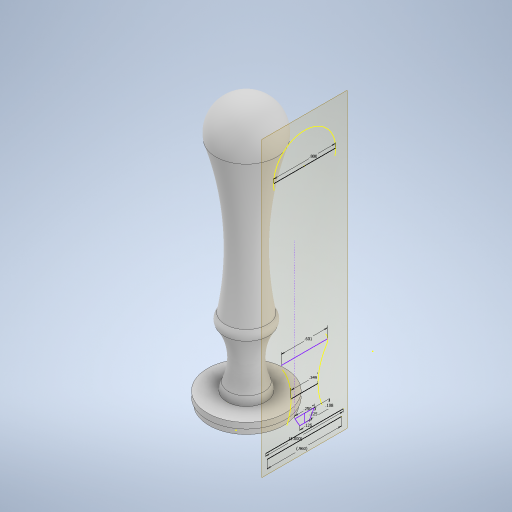
# Autodesk Inventor part: Basic seal 1 full peice
Saved by Autodesk Inventor 2024 (Build 280153000, 153)
## iProperties
Created: 2023-05-18
Part Number: Basic seal 1 full peice
Material: Generic
Document SubType Name: Modeling
Designer: newic
Density: 1 g/cm^3
Appearance: Default
Author: newic
Autodesk Inventor part; units mm, degrees
ref_plane "XZ Plane" through (0, 0, 0) normal (0, 1, 0) x (-1, 0, 0)
ref_plane "XY Plane" through (0, 0, 0) normal (0, 0, 1) x (1, 0, 0)
sketch "Sketch1" plane through (0, 0, 0) normal (0, 1, 0) x (-1, 0, 0)
  circle A0 centre (0, 0) radius 12.7
  line L0 (12.7, 12.7) -> (12.7, -12.7) construction
  line L1 (12.7, -12.7) -> (-12.7, -12.7) construction
  line L2 (-12.7, -12.7) -> (-12.7, 12.7) construction
  line L3 (-12.7, 12.7) -> (12.7, 12.7) construction
  circle A1 centre (0, 0) radius 12.1875
  circle A2 centre (0, 0) radius 11.5722
  line L4 (12.7, 0) -> (-28.224, 0)
  spline S0 degree 4 poles (7.5608, 0) (7.5871, -0.2498) (7.5716, -0.8639) (7.6635, -1.72) (7.771, -2.5827) (7.8796, -3.1444) (8.0283, -3.9996) (8.2528, -4.7367) (8.3389, -5.0369) (8.4927, -5.4299) (8.607, -5.7477) (8.7077, -5.9466) (8.7297, -6.0528) (8.7259, -6.1323) (8.6915, -6.2267) (8.6084, -6.3073) (8.4656, -6.4322) (8.3108, -6.5585) (7.9581, -6.8561) (7.7627, -7.0404) (7.5994, -7.1572) (7.2874, -7.4352) (7.0492, -7.6385) (6.8557, -7.7767) (6.6363, -7.9955) (6.5444, -8.04) (6.425, -8.09) (6.3049, -8.0852) (6.1612, -8.0439) (5.8673, -7.9243) (5.2047, -7.7184) (4.9544, -7.6282) (4.5834, -7.5418) (3.9869, -7.3825) (3.5585, -7.2836) (3.3261, -7.2353) (2.6639, -7.1283) (2.4923, -7.0851) (1.885, -7.0109) (1.2249, -6.9515) (0.9978, -6.9092) (-0.0967, -6.8274) (-0.0908, -6.8879) (-0.9888, -6.8956) (-1.4498, -6.994) (-2.157, -7.03) (-2.8755, -7.1861) (-3.3866, -7.2397) (-4.3934, -7.4794) (-4.8139, -7.612) (-5.3152, -7.7313) (-5.615, -7.8484) (-5.8655, -7.9444) (-6.1746, -8.0443) (-6.2691, -8.0783) (-6.3955, -8.0918) (-6.486, -8.0779) (-6.6705, -8.0058) (-6.661, -7.9168) (-6.8879, -7.7874) (-7.0089, -7.6489) (-7.1824, -7.5178) (-7.3229, -7.3873) (-7.5822, -7.175) (-7.7931, -7.0025) (-8.0826, -6.7466) (-8.2527, -6.613) (-8.4352, -6.4317) (-8.5724, -6.3549) (-8.667, -6.2237) (-8.6858, -6.2037) (-8.7162, -6.092) (-8.7131, -6.0317) (-8.695, -5.9554) (-8.5854, -5.7043) (-8.4697, -5.4626) (-8.3913, -5.2076) (-8.2879, -4.9538) (-8.1958, -4.6121) (-8.0468, -4.045) (-7.9725, -3.8304) (-7.7592, -2.661) (-7.6907, -2.1909) (-7.6151, -1.4373) (-7.564, -0.619) (-7.5516, -0.3428) (-7.5554, -0.0046) (-7.5638, 0) knots 0 0 0 0 0 0.039296 0.055908 0.073069 0.090127 0.10618 0.121509 0.134965 0.146316 0.15619 0.164179 0.170591 0.176443 0.182863 0.190407 0.199969 0.210544 0.221389 0.232964 0.244031 0.25516 0.266564 0.276442 0.284967 0.292352 0.298886 0.30652 0.31685 0.32851 0.341463 0.355682 0.368855 0.381917 0.395666 0.408085 0.420945 0.435034 0.448763 0.464427 0.47884 0.493305 0.508372 0.522986 0.539358 0.555691 0.57306 0.589942 0.605994 0.620829 0.633477 0.645128 0.655027 0.663676 0.671144 0.677933 0.684628 0.692084 0.700281 0.708721 0.71788 0.727519 0.737693 0.74871 0.760009 0.770972 0.781161 0.789961 0.797299 0.803676 0.809144 0.814179 0.820577 0.828361 0.837524 0.847989 0.859019 0.870721 0.882901 0.897625 0.913523 0.930287 0.948149 0.964022 0.978288 1 1 1 1 1
  spline S1 degree 4 poles (7.5608, 0) (7.5871, 0.2498) (7.5716, 0.8639) (7.6635, 1.72) (7.771, 2.5827) (7.8796, 3.1444) (8.0283, 3.9996) (8.2528, 4.7367) (8.3389, 5.0368) (8.4927, 5.4299) (8.607, 5.7477) (8.7077, 5.9466) (8.7297, 6.0528) (8.7259, 6.1323) (8.6915, 6.2267) (8.6084, 6.3073) (8.4656, 6.4322) (8.3108, 6.5585) (7.9581, 6.8561) (7.7627, 7.0404) (7.5994, 7.1572) (7.2874, 7.4352) (7.0492, 7.6385) (6.8557, 7.7767) (6.6363, 7.9955) (6.5444, 8.04) (6.425, 8.09) (6.3049, 8.0852) (6.1612, 8.0439) (5.8673, 7.9243) (5.2047, 7.7184) (4.9544, 7.6282) (4.5834, 7.5418) (3.9869, 7.3825) (3.5585, 7.2836) (3.3261, 7.2353) (2.6639, 7.1283) (2.4923, 7.0851) (1.885, 7.0109) (1.2249, 6.9515) (0.9978, 6.9092) (-0.0967, 6.8274) (-0.0908, 6.8879) (-0.9888, 6.8956) (-1.4498, 6.994) (-2.157, 7.03) (-2.8755, 7.1861) (-3.3866, 7.2397) (-4.3934, 7.4794) (-4.8139, 7.612) (-5.3152, 7.7313) (-5.615, 7.8484) (-5.8655, 7.9444) (-6.1746, 8.0443) (-6.2691, 8.0783) (-6.3955, 8.0918) (-6.486, 8.0779) (-6.6705, 8.0058) (-6.661, 7.9168) (-6.8879, 7.7874) (-7.0089, 7.6489) (-7.1824, 7.5178) (-7.3229, 7.3873) (-7.5822, 7.175) (-7.7931, 7.0025) (-8.0826, 6.7466) (-8.2527, 6.613) (-8.4352, 6.4317) (-8.5724, 6.3549) (-8.667, 6.2237) (-8.6858, 6.2037) (-8.7162, 6.092) (-8.7131, 6.0317) (-8.695, 5.9554) (-8.5854, 5.7043) (-8.4697, 5.4626) (-8.3913, 5.2076) (-8.2879, 4.9538) (-8.1958, 4.6121) (-8.0468, 4.045) (-7.9725, 3.8304) (-7.7592, 2.661) (-7.6907, 2.1909) (-7.6151, 1.4373) (-7.564, 0.619) (-7.5516, 0.3428) (-7.5554, 0.0046) (-7.5638, 0) knots 0 0 0 0 0 0.039296 0.055908 0.073069 0.090127 0.10618 0.121509 0.134965 0.146316 0.15619 0.164179 0.170591 0.176443 0.182863 0.190407 0.199969 0.210544 0.221389 0.232964 0.244031 0.25516 0.266564 0.276442 0.284967 0.292352 0.298886 0.30652 0.31685 0.32851 0.341463 0.355682 0.368855 0.381917 0.395666 0.408085 0.420945 0.435034 0.448763 0.464427 0.47884 0.493305 0.508372 0.522986 0.539358 0.555691 0.57306 0.589942 0.605994 0.620829 0.633477 0.645128 0.655027 0.663676 0.671144 0.677933 0.684628 0.692084 0.700281 0.708721 0.71788 0.727519 0.737693 0.74871 0.760009 0.770972 0.781161 0.789961 0.797299 0.803676 0.809144 0.814179 0.820577 0.828361 0.837524 0.847989 0.859019 0.870721 0.882901 0.897625 0.913523 0.930287 0.948149 0.964022 0.978288 1 1 1 1 1
  spline S2 degree 4 poles (6.6698, 0) (6.6871, -0.3978) (6.6713, -0.7815) (6.7409, -1.5229) (6.8536, -2.5936) (6.9252, -2.906) (7.0997, -3.8444) (7.2267, -4.3825) (7.3633, -4.7956) (7.4896, -5.3512) (7.6112, -5.5391) (7.6677, -5.7689) (7.6975, -5.7897) (7.7062, -5.8965) (7.6285, -5.9815) (7.572, -6.0514) (7.3996, -6.178) (7.1331, -6.4178) (6.9588, -6.5681) (6.6364, -6.8323) (6.5004, -6.9541) (6.3704, -7.0647) (6.3037, -7.1086) (6.2234, -7.1388) (6.1631, -7.1283) (6.0268, -7.0924) (5.9076, -7.0514) (5.5806, -6.952) (5.3855, -6.8908) (5.038, -6.812) (4.9484, -6.7624) (4.2814, -6.6028) (4.0156, -6.5429) (3.8882, -6.5183) (3.3037, -6.3965) (2.8824, -6.3286) (2.5502, -6.2731) (2.4025, -6.2241) (1.6246, -6.1518) (1.37, -6.0874) (1.1134, -6.1) (0.6072, -6.0267) (0.5913, -6.054) (0.1833, -6.0225) (0.0815, -6.0123) (-0.2846, -6.0335) (-0.5883, -6.0362) (-0.9225, -6.0806) (-1.3996, -6.1121) (-1.6329, -6.1378) (-2.1126, -6.197) (-2.4639, -6.2503) (-2.782, -6.3007) (-3.1586, -6.3702) (-3.2077, -6.3787) (-3.7538, -6.4818) (-4.0918, -6.5436) (-4.3482, -6.6242) (-4.8814, -6.7303) (-5.2054, -6.8556) (-5.5087, -6.9063) (-5.6572, -6.9822) (-5.9526, -7.0706) (-6.1139, -7.1317) (-6.1762, -7.1269) (-6.2789, -7.1205) (-6.425, -7.0257) (-6.5484, -6.9167) (-6.706, -6.7703) (-6.9687, -6.5457) (-7.0919, -6.4669) (-7.3885, -6.1958) (-7.4865, -6.1263) (-7.6283, -5.9822) (-7.6822, -5.9316) (-7.7081, -5.8596) (-7.7006, -5.7637) (-7.6112, -5.6344) (-7.5282, -5.3549) (-7.4652, -5.1836) (-7.3295, -4.7829) (-7.1819, -4.1547) (-7.1117, -3.848) (-6.9524, -3.2013) (-6.8781, -2.6524) (-6.8463, -2.4403) (-6.7659, -1.8396) (-6.735, -1.4493) (-6.7089, -1.1731) (-6.6784, -0.6337) (-6.6716, -0.3941) (-6.6731, -0.0474) (-6.6763, 0) knots 0 0 0 0 0 0.039448 0.055349 0.072269 0.088737 0.104506 0.120552 0.134467 0.146293 0.155548 0.162505 0.168442 0.174025 0.180717 0.189099 0.198791 0.210185 0.221737 0.232089 0.240921 0.247815 0.253612 0.259204 0.265359 0.273108 0.282299 0.292472 0.302955 0.314654 0.326295 0.337305 0.349803 0.361846 0.37389 0.386284 0.399242 0.411449 0.423896 0.437159 0.44785 0.458402 0.468238 0.477683 0.488335 0.499312 0.51153 0.523717 0.536339 0.54908 0.561517 0.573881 0.584661 0.595665 0.606838 0.61814 0.631344 0.644301 0.656608 0.668396 0.679342 0.688982 0.697238 0.704622 0.711137 0.717919 0.725945 0.735426 0.745345 0.756153 0.766663 0.776344 0.78489 0.791619 0.7976 0.803458 0.810655 0.819014 0.829148 0.841433 0.854403 0.869138 0.884301 0.898105 0.912368 0.925751 0.938316 0.951323 0.9634 0.975086 1 1 1 1 1
  spline S3 degree 4 poles (6.6698, 0) (6.6871, 0.3978) (6.6713, 0.7814) (6.7409, 1.5229) (6.8536, 2.5936) (6.9252, 2.906) (7.0997, 3.8444) (7.2267, 4.3825) (7.3633, 4.7956) (7.4896, 5.3512) (7.6112, 5.5391) (7.6677, 5.7689) (7.6975, 5.7897) (7.7062, 5.8965) (7.6285, 5.9815) (7.572, 6.0514) (7.3996, 6.178) (7.1331, 6.4178) (6.9588, 6.5681) (6.6364, 6.8323) (6.5004, 6.9541) (6.3704, 7.0646) (6.3037, 7.1085) (6.2234, 7.1388) (6.1631, 7.1283) (6.0268, 7.0924) (5.9076, 7.0514) (5.5806, 6.952) (5.3855, 6.8908) (5.038, 6.812) (4.9484, 6.7624) (4.2814, 6.6028) (4.0156, 6.5429) (3.8882, 6.5183) (3.3037, 6.3965) (2.8824, 6.3286) (2.5502, 6.2731) (2.4025, 6.2241) (1.6246, 6.1517) (1.37, 6.0874) (1.1134, 6.1) (0.6072, 6.0267) (0.5913, 6.054) (0.1833, 6.0225) (0.0815, 6.0123) (-0.2846, 6.0335) (-0.5883, 6.0362) (-0.9225, 6.0806) (-1.3996, 6.1121) (-1.6329, 6.1378) (-2.1126, 6.197) (-2.4639, 6.2503) (-2.782, 6.3007) (-3.1586, 6.3702) (-3.2077, 6.3787) (-3.7538, 6.4818) (-4.0918, 6.5436) (-4.3482, 6.6242) (-4.8814, 6.7303) (-5.2054, 6.8556) (-5.5087, 6.9063) (-5.6572, 6.9822) (-5.9526, 7.0706) (-6.1139, 7.1317) (-6.1762, 7.1269) (-6.2789, 7.1205) (-6.425, 7.0257) (-6.5484, 6.9166) (-6.706, 6.7703) (-6.9687, 6.5457) (-7.0919, 6.4669) (-7.3885, 6.1958) (-7.4865, 6.1263) (-7.6283, 5.9822) (-7.6822, 5.9316) (-7.7081, 5.8596) (-7.7006, 5.7637) (-7.6112, 5.6344) (-7.5282, 5.3549) (-7.4652, 5.1836) (-7.3295, 4.7829) (-7.1819, 4.1547) (-7.1117, 3.848) (-6.9524, 3.2013) (-6.8781, 2.6524) (-6.8463, 2.4403) (-6.7659, 1.8396) (-6.735, 1.4493) (-6.7089, 1.1731) (-6.6784, 0.6337) (-6.6716, 0.3941) (-6.6731, 0.0474) (-6.6763, 0) knots 0 0 0 0 0 0.039448 0.055349 0.072269 0.088737 0.104506 0.120552 0.134467 0.146293 0.155548 0.162505 0.168442 0.174025 0.180717 0.189099 0.198791 0.210185 0.221737 0.232089 0.240921 0.247815 0.253612 0.259204 0.265359 0.273108 0.282299 0.292472 0.302955 0.314654 0.326295 0.337305 0.349803 0.361846 0.37389 0.386284 0.399242 0.411449 0.423896 0.437159 0.44785 0.458402 0.468238 0.477683 0.488335 0.499312 0.51153 0.523717 0.536339 0.54908 0.561517 0.573881 0.584661 0.595665 0.606838 0.61814 0.631344 0.644301 0.656608 0.668396 0.679342 0.688982 0.697238 0.704622 0.711137 0.717919 0.725945 0.735426 0.745345 0.756153 0.766663 0.776344 0.78489 0.791619 0.7976 0.803458 0.810655 0.819014 0.829148 0.841433 0.854403 0.869138 0.884301 0.898105 0.912368 0.925751 0.938316 0.951323 0.9634 0.975086 1 1 1 1 1
  line L5 (1.0941, 0) -> (1.0941, -2.0952)
  line L6 (1.0941, -2.0952) -> (3.9049, -2.2474)
  line L7 (3.9049, -2.2474) -> (4.7904, -1.5612)
  line L8 (-0.5884, 0) -> (-0.5898, -1.9938)
  line L9 (-0.5898, -1.9938) -> (-4.3298, -1.7894)
  line L10 (-4.3298, -1.7894) -> (-5.2324, -1.0809)
  line L11 (5.0927, -1.7005) -> (5.1051, -4.9152)
  line L12 (4.7853, -5.0014) -> (3.8243, -3.9243)
  line L13 (3.8243, -3.9243) -> (-4.2884, -3.485)
  line L14 (-4.2884, -3.485) -> (-5.2324, -4.5455)
  line L15 (-5.5377, -4.4469) -> (-5.5322, -1.2345)
  arc A3 (5.0927, -1.7005) -> (4.7904, -1.5612) centre (4.931, -1.6537) ccw
  arc A4 (4.7853, -5.0014) -> (5.1051, -4.9152) centre (4.9338, -4.9158) ccw
  arc A5 (-5.5377, -4.4469) -> (-5.2324, -4.5455) centre (-5.3693, -4.4472) ccw
  arc A6 (-5.2324, -1.0809) -> (-5.5322, -1.2345) centre (-5.368, -1.1857) ccw
  line L16 (1.0941, 0) -> (1.0941, 2.0952)
  line L17 (1.0941, 2.0952) -> (3.9049, 2.2474)
  line L18 (3.9049, 2.2474) -> (4.7904, 1.5612)
  line L19 (-0.5884, 0) -> (-0.5898, 1.9938)
  line L20 (-0.5898, 1.9938) -> (-4.3298, 1.7894)
  line L21 (-4.3298, 1.7894) -> (-5.2324, 1.0809)
  line L22 (5.0927, 1.7005) -> (5.1051, 4.9152)
  line L23 (4.7853, 5.0014) -> (3.8243, 3.9243)
  line L24 (3.8243, 3.9243) -> (-4.2884, 3.485)
  line L25 (-4.2884, 3.485) -> (-5.2324, 4.5455)
  arc A7 (4.7904, 1.5612) -> (5.0927, 1.7005) centre (4.931, 1.6537) ccw
  arc A8 (5.1051, 4.9152) -> (4.7853, 5.0014) centre (4.9338, 4.9158) ccw
  arc A9 (-5.2324, 4.5455) -> (-5.5377, 4.4469) centre (-5.3693, 4.4472) ccw
  arc A10 (-5.5322, 1.2345) -> (-5.2324, 1.0809) centre (-5.368, 1.1857) ccw
  line L26 (-5.5377, 4.4469) -> (-5.5322, 1.2345)
  point P0 (7.582, -0.4475)
  point P1 (7.6181, -1.1897)
  point P2 (7.6938, -1.9478)
  point P3 (7.7753, -2.5562)
  point P4 (7.8781, -3.1491)
  point P5 (8.0672, -4.0731)
  point P6 (8.2624, -4.7725)
  point P7 (8.3673, -5.0974)
  point P8 (8.5065, -5.4722)
  point P9 (8.6396, -5.8063)
  point P10 (8.7107, -5.9813)
  point P11 (8.7259, -6.0648)
  point P12 (8.7208, -6.1314)
  point P13 (8.6916, -6.2086)
  point P14 (8.625, -6.2893)
  point P15 (8.5035, -6.398)
  point P16 (8.3259, -6.5472)
  point P17 (7.9666, -6.8536)
  point P18 (7.7597, -7.0347)
  point P19 (7.5972, -7.1666)
  point P20 (7.2997, -7.4223)
  point P21 (7.0358, -7.6431)
  point P22 (6.8133, -7.8257)
  point P23 (6.615, -7.9971)
  point P24 (6.5232, -8.0478)
  point P25 (6.4269, -8.0794)
  point P26 (6.3307, -8.0824)
  point P27 (6.2157, -8.0568)
  point P28 (5.939, -7.9581)
  point P29 (5.2485, -7.7291)
  point P30 (4.9341, -7.6303)
  point P31 (4.5863, -7.5395)
  point P32 (3.9767, -7.3836)
  point P33 (3.5714, -7.2881)
  point P34 (3.2721, -7.2292)
  point P35 (2.7391, -7.1371)
  point P36 (2.4628, -7.0879)
  point P37 (1.9303, -7.0199)
  point P38 (1.3001, -6.9537)
  point P39 (0.8618, -6.905)
  point P40 (0.0288, -6.8555)
  point P41 (-0.2052, -6.8728)
  point P42 (-0.8545, -6.91)
  point P43 (-1.4645, -6.978)
  point P44 (-2.1388, -7.0515)
  point P45 (-2.824, -7.1641)
  point P46 (-3.4525, -7.2709)
  point P47 (-4.4053, -7.4924)
  point P48 (-4.9149, -7.6324)
  point P49 (-5.3455, -7.7526)
  point P50 (-5.6379, -7.8568)
  point P51 (-5.9277, -7.9626)
  point P52 (-6.1933, -8.0512)
  point P53 (-6.2931, -8.0776)
  point P54 (-6.3884, -8.0863)
  point P55 (-6.4903, -8.0706)
  point P56 (-6.6308, -8.0034)
  point P57 (-6.6877, -7.9317)
  point P58 (-6.8516, -7.7973)
  point P59 (-7.0164, -7.6529)
  point P60 (-7.1659, -7.5263)
  point P61 (-7.3162, -7.3971)
  point P62 (-7.5527, -7.1992)
  point P63 (-7.8063, -6.9879)
  point P64 (-8.0883, -6.7461)
  point P65 (-8.2789, -6.5822)
  point P66 (-8.4597, -6.4263)
  point P67 (-8.5958, -6.3127)
  point P68 (-8.6662, -6.2262)
  point P69 (-8.6877, -6.1869)
  point P70 (-8.71, -6.101)
  point P71 (-8.7118, -6.043)
  point P72 (-8.6987, -5.9829)
  point P73 (-8.6117, -5.7675)
  point P74 (-8.4802, -5.4672)
  point P75 (-8.3902, -5.2184)
  point P76 (-8.3037, -4.977)
  point P77 (-8.2036, -4.6385)
  point P78 (-8.0738, -4.1578)
  point P79 (-7.9798, -3.7988)
  point P80 (-7.7876, -2.7953)
  point P81 (-7.688, -2.1188)
  point P82 (-7.614, -1.3524)
  point P83 (-7.5689, -0.6701)
  point P84 (-7.5559, -0.2905)
  point P85 (-7.5591, -0.0322)
  point P86 (7.582, 0.4475)
  point P87 (7.6181, 1.1897)
  point P88 (7.6938, 1.9478)
  point P89 (7.7753, 2.5562)
  point P90 (7.8781, 3.1491)
  point P91 (8.0672, 4.0731)
  point P92 (8.2624, 4.7725)
  point P93 (8.3673, 5.0973)
  point P94 (8.5065, 5.4722)
  point P95 (8.6396, 5.8063)
  point P96 (8.7107, 5.9813)
  point P97 (8.7259, 6.0648)
  point P98 (8.7208, 6.1314)
  point P99 (8.6916, 6.2085)
  point P100 (8.625, 6.2893)
  point P101 (8.5035, 6.398)
  point P102 (8.3259, 6.5472)
  point P103 (7.9666, 6.8536)
  point P104 (7.7597, 7.0347)
  point P105 (7.5972, 7.1666)
  point P106 (7.2997, 7.4223)
  point P107 (7.0358, 7.6431)
  point P108 (6.8133, 7.8257)
  point P109 (6.615, 7.997)
  point P110 (6.5232, 8.0478)
  point P111 (6.4269, 8.0794)
  point P112 (6.3307, 8.0824)
  point P113 (6.2157, 8.0568)
  point P114 (5.939, 7.9581)
  point P115 (5.2485, 7.7291)
  point P116 (4.9341, 7.6303)
  point P117 (4.5863, 7.5395)
  point P118 (3.9767, 7.3836)
  point P119 (3.5714, 7.2881)
  point P120 (3.2721, 7.2292)
  point P121 (2.7391, 7.1371)
  point P122 (2.4628, 7.0879)
  point P123 (1.9303, 7.0199)
  point P124 (1.3001, 6.9537)
  point P125 (0.8618, 6.905)
  point P126 (0.0288, 6.8555)
  point P127 (-0.2052, 6.8727)
  point P128 (-0.8545, 6.91)
  point P129 (-1.4645, 6.978)
  point P130 (-2.1388, 7.0515)
  point P131 (-2.824, 7.1641)
  point P132 (-3.4525, 7.2709)
  point P133 (-4.4053, 7.4924)
  point P134 (-4.9149, 7.6324)
  point P135 (-5.3455, 7.7526)
  point P136 (-5.6379, 7.8568)
  point P137 (-5.9277, 7.9626)
  point P138 (-6.1933, 8.0512)
  point P139 (-6.2931, 8.0776)
  point P140 (-6.3884, 8.0863)
  point P141 (-6.4903, 8.0706)
  point P142 (-6.6308, 8.0034)
  point P143 (-6.6877, 7.9317)
  point P144 (-6.8516, 7.7973)
  point P145 (-7.0164, 7.6529)
  point P146 (-7.1659, 7.5263)
  point P147 (-7.3162, 7.3971)
  point P148 (-7.5527, 7.1992)
  point P149 (-7.8063, 6.9879)
  point P150 (-8.0883, 6.746)
  point P151 (-8.2789, 6.5822)
  point P152 (-8.4597, 6.4263)
  point P153 (-8.5958, 6.3127)
  point P154 (-8.6662, 6.2262)
  point P155 (-8.6877, 6.1869)
  point P156 (-8.71, 6.101)
  point P157 (-8.7118, 6.043)
  point P158 (-8.6987, 5.9829)
  point P159 (-8.6117, 5.7675)
  point P160 (-8.4802, 5.4672)
  point P161 (-8.3902, 5.2183)
  point P162 (-8.3037, 4.977)
  point P163 (-8.2036, 4.6385)
  point P164 (-8.0738, 4.1578)
  point P165 (-7.9798, 3.7987)
  point P166 (-7.7876, 2.7953)
  point P167 (-7.688, 2.1188)
  point P168 (-7.614, 1.3524)
  point P169 (-7.5689, 0.6701)
  point P170 (-7.5559, 0.2905)
  point P171 (-7.5591, 0.0322)
  point P172 (6.6836, -0.5412)
  point P173 (6.7072, -1.0761)
  point P174 (6.774, -1.8261)
  point P175 (6.8568, -2.5341)
  point P176 (6.9346, -2.9728)
  point P177 (7.1026, -3.8229)
  point P178 (7.2446, -4.4136)
  point P179 (7.3804, -4.8955)
  point P180 (7.5322, -5.3935)
  point P181 (7.6322, -5.6381)
  point P182 (7.6779, -5.7675)
  point P183 (7.6936, -5.8064)
  point P184 (7.6937, -5.8803)
  point P185 (7.6435, -5.9655)
  point P186 (7.5821, -6.0322)
  point P187 (7.446, -6.1471)
  point P188 (7.1705, -6.3831)
  point P189 (6.9233, -6.5957)
  point P190 (6.6151, -6.8536)
  point P191 (6.4599, -6.9878)
  point P192 (6.3548, -7.0726)
  point P193 (6.2905, -7.111)
  point P194 (6.2287, -7.1307)
  point P195 (6.1718, -7.1283)
  point P196 (6.068, -7.1023)
  point P197 (5.9271, -7.0591)
  point P198 (5.6207, -6.9639)
  point P199 (5.36, -6.8886)
  dimension "d0" = 25.4
  dimension "d32" = 25.4
  dimension "d39" = 25.4
  constraints: 195 symmetric about line, 46 end point, 17 point on circle, 11 centre point, 6 point on line, 3 coincident, 2 tangent, 1 horizontal, 1 midpoint, 1 perpendicular, 368 other
  measures "d0" diameter of A0
  measures "d32" distance of L2.end L0.start
  measures "d39" distance of L0.start L0.end
extrude "Extrusion1" add sketch "Sketch1" along normal blind 1.905 contours L4 A2 A1 | A1 L4 A2 | S0 L4 S2 | L4 S3 S1 | L5 L6 L7 A3 L11 A4 L12 L13 L14 A5 L15 A6 L10 L9 L8 L4 | L4 L19 L20 L21 A10 L26 A9 L25 L24 L23 A8 L22 A7 L18 L17 L16
sketch "Sketch2" plane through (0, 1.905, 0) normal (0, 1, 0) x (1, 0, 0)
  line L0 (12.7067, 12.7) -> (12.7067, -12.7) construction
  line L1 (12.7067, -12.7) -> (-12.6933, -12.7) construction
  line L2 (-12.6933, -12.7) -> (-12.6933, 12.7) construction
  line L3 (-12.6933, 12.7) -> (12.7067, 12.7) construction
  circle A0 centre (0, 0) radius 12.1875 projected
  line L4 (-12.1875, 0) -> (-18.0724, 0)
  circle A1 centre (0, 0) radius 12.7
  dimension "d92" = 25.4
  dimension "d98" = 25.4
  constraints: 2 end point, 1 centre point, 1 coincident, 1 horizontal, 1 horizontal alignment, 3 other
  measures "d92" distance of L2.end L0.start
  measures "d98" diameter of A1
extrude "Extrusion2" add sketch "Sketch2" along normal blind 1.905 contours A0 | A1
sketch "Sketch3" plane through (0, 0, 0) normal (0, 0, 1) x (1, 0, 0)
  line L0 (0, 0) -> (0, 88.9)
  line L1 (134.3126, 257.1223) -> (473.4262, 257.1223) construction
  line L2 (473.4262, 257.1223) -> (473.4262, 17.1036) construction
  line L3 (473.4262, 17.1036) -> (134.3126, 17.1036) construction
  line L4 (134.3126, 17.1036) -> (134.3126, 257.1223) construction
  circle A0 centre (112.6944, 39.6279) radius 12.7
  circle A1 centre (0, 44.45) radius 5.08
  circle A2 centre (0, 77.1578) radius 10.16
  line L5 (0, 44.45) -> (0, 3.81)
  line L6 (12.7, 3.81) -> (-12.7, 3.81) projected
  circle A3 centre (0, 24.13) radius 5.08
  circle A4 centre (5.0788, 24.2425) radius 2.54
  circle A5 centre (-4.9792, 23.1233) radius 2.54
  line L7 (-4.9792, 23.1233) -> (-13.9595, 32.1035)
  line L8 (-4.9792, 23.1233) -> (7.7208, 23.1233) construction
  line L9 (5.0788, 24.2425) -> (14.059, 33.2227)
  line L10 (5.0788, 24.2425) -> (17.7788, 24.2425) construction
  line L11 (5.0788, 24.2425) -> (12.9329, 19.8885)
  line L12 (-4.9792, 23.1233) -> (-13.9595, 14.143)
  line L13 (-4.9792, 23.1233) -> (7.7208, 23.1233) construction
  arc A6 (9.9682, 75.1929) -> (6.8748, 26.0385) centre (108.777, 44.3001) ccw
  arc A7 (-6.7753, 24.9193) -> (-9.9499, 75.1021) centre (-109.0911, 43.6386) ccw
  circle A8 centre (0, 3.81) radius 6.35
  line L14 (0, 24.13) -> (0, 3.81)
  circle A9 centre (0, 13.97) radius 4.445
  arc A10 (-6.35, 3.81) -> (-6.7753, 21.3272) centre (-23.0464, 12.1684) ccw
  arc A11 (7.3002, 23.011) -> (5.779, 6.4416) centre (22.4276, 13.2676) ccw
  point P0 (0, 87.3178)
  point P1 (0, 3.81)
  point P2 (6.35, 3.81)
  dimension "d101" = 88.9
  dimension "d103" = 25.4
  dimension "d118" = 10.16
  dimension "d122" = 20.32
  dimension "d123" = 10.16
  dimension "d124" = 5.08
  dimension "d125" = 5.08
  dimension "d126" = 12.7
  dimension "d127" = 135
  dimension "d128" = 12.7
  dimension "d129" = 45
  dimension "d130" = 12.7
  dimension "d131" = 135
  dimension "d132" = 12.7
  dimension "d133" = 8.89
  constraints: 20 end point, 18 point on circle, 12 centre point, 6 point on line, 4 midpoint, 3 equal length, 3 horizontal, 3 tangent, 1 coincident, 1 collinear, 1 vertical, 2 other
  measures "d101" distance of L0.start L0.end
  measures "d103" diameter of A0
  measures "d118" diameter of A1
  measures "d122" diameter of A2
  measures "d123" diameter of A3
  measures "d124" diameter of A4
  measures "d125" diameter of A5
  measures "d126" distance of L7.start L7.end
  measures "d127" angle of L8 L7
  measures "d128" distance of L9.start L9.end
  measures "d129" angle of L10 L9
  measures "d130" distance of L7.start L12.end
  measures "d131" angle of L12 L13
  measures "d132" diameter of A8
  measures "d133" diameter of A9
revolve "Revolution1" add sketch "Sketch3" angle 360 about axis through (0, 44.45, 0) along (0, -1, 0) picked at (0.2042, 9.7508) picked at (0.3297, 15.6262) picked at (3.3442, 44.0732) contours L0 A9 A8 L6 | L0 A8 A9 | L0 A9 A8 | A9 A11 A8 | L0 A3 A4 A11 A9 | L0 A3 A4 | A4 A3 L11 A11 | A4 A3 | L11 L9 A4 | L0 A1 A2 A6 A4 A3 | A4 L9 A3 | L0 A1 | A2 L0 A6
sketch "Sketch4" plane through (0, 0, 0) normal (1, 0, 0) x (0, 1, 0)
  line L0 (3.81, 6.35) -> (3.81, -6.35) projected
  line L1 (3.81, 2.8038) -> (6.4416, 4.0782)
  line L2 (6.4416, 5.779) -> (6.4416, -5.779) projected
  line L3 (3.81, 0) -> (6.4416, 0)
  line L4 (6.4416, 4.0782) -> (6.4416, 0)
  line L5 (3.81, -2.8038) -> (6.4416, -4.0782)
  line L6 (6.4416, -5.779) -> (6.4416, 5.779)
  point P0 (0, 0)
  constraints: 10 end point, 4 symmetric about line, 3 point on line, 1 horizontal, 1 perpendicular
ref_plane "Work Plane1" through (19.05, 0, 0) normal (1, 0, 0) x (0, 1, 0)
sketch "Sketch5" plane through (19.05, 0, 0) normal (1, 0, 0) x (0, 1, 0)
  line L0 (4.2354, -1.5875) -> (4.2354, 1.5875)
  line L1 (6.985, 3.175) -> (6.985, -3.175)
  line L2 (4.2354, -1.5875) -> (4.2354, 1.5875)
  line L3 (6.985, 3.175) -> (57.785, 3.175) construction
  line L4 (6.985, -3.175) -> (4.2354, -1.5875)
  line L5 (6.985, 3.175) -> (4.2354, 1.5875)
  line L6 (24.3714, 7.6504) -> (24.3714, -7.6155)
  arc A0 (23.011, -7.3002) -> (26.0385, -6.8748) centre (24.2425, -5.0788) ccw projected
  line L7 (0, -12.1875) -> (0, 12.1875) projected
  line L8 (0, 12.1875) -> (0, -12.1875)
  line L9 (1.905, -12.7) -> (1.905, 12.7) projected
  line L10 (1.905, 12.7) -> (1.905, -12.7)
  arc A1 (6.4416, 5.779) -> (23.011, 7.3002) centre (13.2676, 22.4276) ccw projected
  line L11 (13.2676, 4.434) -> (13.2676, -4.434)
  arc A2 (23.011, -7.3002) -> (6.4416, -5.779) centre (13.2676, -22.4276) ccw projected
  arc A3 (75.1929, -9.9682) -> (75.1929, 9.9682) centre (77.1578, 0) ccw projected
  line L12 (77.226, 10.1598) -> (77.226, -10.1598)
  line L13 (4.2354, 0) -> (6.985, 0)
  dimension "d139" = 3.175
  dimension "d142" = 3.175
  dimension "d143" = 24.375
  dimension "d144" = 25.4
  dimension "d145" = 15.2658
  dimension "d146" = 8.868
  dimension "d147" = 6.35
  dimension "d148" = 20.3195
  dimension "d149" = 2.7496
  constraints: 24 end point, 5 point on circle, 3 vertical, 2 collinear, 2 midpoint, 1 horizontal, 1 parallel
  measures "d139" distance of L1.end L0.start
  measures "d142" distance of L0.start L0.end
  measures "d143" distance of L7.start L7.end
  measures "d144" distance of L9.start L9.end
  measures "d145" distance of L6.start L6.end
  measures "d146" distance of L11.start L11.end
  measures "d147" distance of L1.start L1.end
  measures "d148" distance of L12.start L12.end
  measures "d149" distance of L13.start L13.end
body "Solid1"
